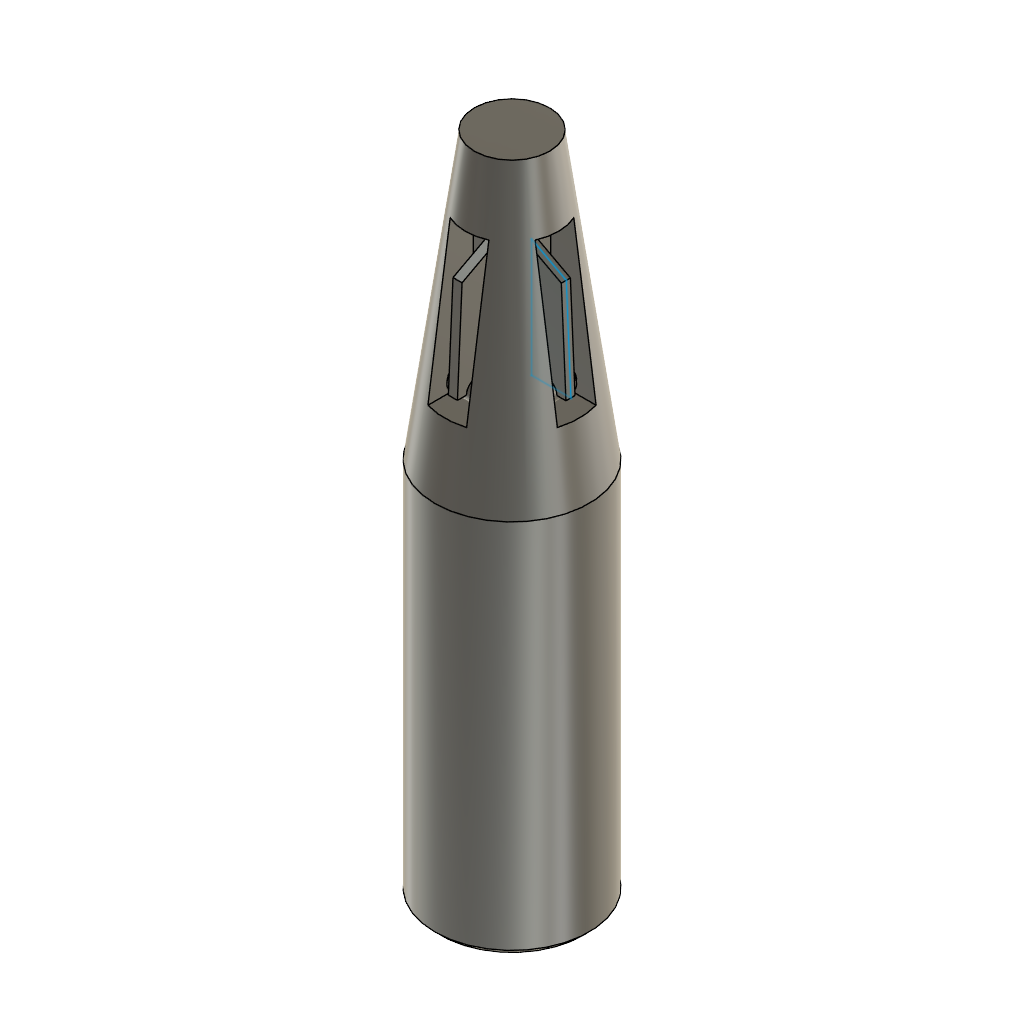
Canard Actuation Assembly (Autodesk Fusion 360 archive; units mm, degrees)
design "Canard Actuation Assembly"
part number: 2026-09-10-19-23-54-107
part number: 2026-09-14-21-49-10-628
part number: 2026-09-14-21-49-10-651
part number: 2026-09-14-21-49-10-660
part number: 2026-09-14-21-49-10-667
part number: 2026-09-14-21-49-10-675
part number: 2026-09-14-21-49-10-684
part number: 2026-09-14-21-49-10-692
part number: 2026-09-14-21-49-10-700
part number: 2026-09-14-21-49-10-708
Autodesk Fusion 360 part; units mm, degrees
note: some values were not read from the file. Chosen so that the rebuilt part matches the saved one: which bodies a step acts on.
sketch "Sketch1" plane through (0, 0, 0) normal (1, 0, 0) x (0, 1, 0)
  line L0 (0, 0) -> (0, -124.7)
  line L1 (0, -124.7) -> (25.5, -124.7)
  line L2 (25.5, -124.7) -> (25.5, 0)
  line L3 (25.5, 0) -> (12.465, 94.3539)
  line L4 (12.465, 94.3539) -> (0, 94.3539)
  line L5 (0, 94.3539) -> (0, 0)
  dimension "d5" = 124.7
  dimension "d6" = 25.5
  dimension "d7" = 124.7
  dimension "d8" = 95.25
  constraint coincident L0.start L5.end
  constraint vertical L0
  constraint perpendicular L0 L1
  constraint perpendicular L1 L2
  constraint horizontal L4
  constraint perpendicular L4 L5
  measures "d5" distance of L0.start L0.end
  measures "d6" distance of L0.end L1.end
  measures "d7" distance of L1.end L2.end
  measures "d8" distance of L2.end L3.end
revolve "Revolve1" add sketch "Sketch1" angle 360 about axis through (0, 0, 0) along (0, 0, -1) makes body 1
sketch "Sketch2" plane through (0, 0, 0) normal (0, 1, 0) x (1, 0, 0)
  line L0 (-6.3965, -72.9001) -> (5.4277, -72.9001)
  line L1 (5.4277, -72.9001) -> (5.4277, -22.9001)
  line L2 (5.4277, -22.9001) -> (-6.3965, -22.9001)
  line L3 (-6.3965, -22.9001) -> (-6.3965, -72.9001)
  dimension "d10" = 50
  constraint horizontal L0
  constraint vertical L1
  constraint horizontal L2
  constraint vertical L3
  measures "d10" distance of L0.start L2.end
extrude "Extrude1" cut sketch "Sketch2" along normal mid plane 60 bodies 1
pattern_circular "C-Pattern1" count 4 over 360 about axis through (0, 0, 0) along (0, 0, -1) of "Extrude1"
sketch "Sketch4" plane through (0, 0, 0) normal (0, 1, 0) x (1, 0, 0)
  line L0 (6.455, -27.1919) -> (6.455, -66.1919)
  line L1 (6.455, -66.1919) -> (17.9112, -60.1005)
  line L2 (17.9112, -60.1005) -> (19.4375, -27.1919)
  line L3 (19.4375, -27.1919) -> (6.455, -27.1919)
  dimension "d16" = 39
  dimension "d17" = 62
  constraint vertical L0
  constraint perpendicular L0 L3
  measures "d16" distance of L0.start L0.end
  measures "d17" angle of L0 L1
extrude "Extrude2" add sketch "Sketch4" along normal mid plane 3 separate body makes body 2
sketch "Sketch6" plane through (0, 0, 0) normal (0, 1, 0) x (1, 0, 0)
  line L0 (17.4442, -27.1976) -> (12.9542, -27.1976)
  circle A0 centre (12.9542, -27.1976) radius 3.5
  dimension "d25" = 4.49
  dimension "d26" = 7
  constraint horizontal L0
  constraint coincident L0.end A0.centre
  measures "d25" distance of L0.start L0.end
  measures "d26" diameter of A0
extrude "Extrude4" add sketch "Sketch6" along normal mid plane 10 bodies 2
chamfer "Chamfer1" distance 2 angle 45 1 faces at (-6.6456, 4.0293, -124.7) on bodies 1
sketch "Sketch9" plane through (0, -5, 0) normal (0, -1, 0) x (1, 0, 0)
  circle A0 centre (12.9542, 27.1976) radius 3.5
  circle A1 centre (12.9542, 27.1976) radius 1.5
  dimension "d44" = 3
  constraint concentric A0 A1
  measures "d44" diameter of A1
extrude "Extrude7" add sketch "Sketch9" along normal blind 4 and the other way blind 14 separate body contours A1 makes body 3
sketch "Sketch10" plane through (0, -5, 0) normal (0, -1, 0) x (1, 0, 0)
  circle A0 centre (12.9542, 27.1976) radius 3.5
  circle A1 centre (12.9542, 27.1976) radius 2
  dimension "d49" = 4
  constraint concentric A0 A1
  measures "d49" diameter of A1
pattern_circular "C-Pattern5" count 4 over 360 about axis through (0, 0, 0) along (0, 0, -1) of bodies 2 3 makes body 4 at (-1.5, -12.0128, 52.2489) makes body 5 at (-12.0128, 1.5, 52.2489) makes body 6 at (1.5, 12.0128, 52.2489) makes body 7 at (4.3333, -11.4617, 27.0482) makes body 8 at (-14.4468, -4.3333, 27.0482) makes body 9 at (0.3333, 14.4524, 27.1228)
sketch "Sketch12" plane through (-9, 0, 0) normal (-1, 0, 0) x (0, -1, 0)
  circle A0 centre (12.9542, 27.1976) radius 1.5
  circle A1 centre (12.9542, 27.1976) radius 2
  dimension "d61" = 4
  constraint concentric A0 A1
  measures "d61" diameter of A1
extrude "Extrude11" cut sketch "Sketch12" along normal blind 0 and the other way blind 24 bodies 1
pattern_circular "C-Pattern6" count 4 over 360 about axis through (0, 0, 0) along (0, 0, -1) of "Extrude11"
copy_body "Body->Comp1" bodies 1 removing the originals makes body 10 in component "Component"
copy_body "Body->Comp2" bodies 2 removing the originals makes body 11 in component "Canard_Fin1"
copy_body "Body->Comp3" bodies 4 removing the originals makes body 12 in component "Canard_Fin1 (1)"
copy_body "Body->Comp4" bodies 5 removing the originals makes body 13 in component "Canard_Fin1 (2)"
copy_body "Body->Comp5" bodies 3 removing the originals makes body 14 in component "Hinge_Pin1"
copy_body "Body->Comp6" bodies 9 removing the originals makes body 15 in component "Hinge_Pin4"
copy_body "Body->Comp7" bodies 6 removing the originals makes body 16 in component "Canard_Fin1 (3)"
copy_body "Body->Comp8" bodies 8 removing the originals makes body 17 in component "Hinge_Pin3"
copy_body "Body->Comp9" bodies 7 removing the originals makes body 18 in component "Hinge_Pin2"
component "Component" placed x (1, 0, 0) y (0, 1, 0) z (0, 0, 1) at (0, 0, 0)
component "Canard_Fin1" placed x (1, 0, 0) y (0, 1, 0) z (0, 0, 1) at (0, -0.1035, 0)
component "Canard_Fin1 (1)" placed x (1, 0, 0) y (0, 1, 0) z (0, 0, 1) at (-0.1035, 0, 0)
component "Canard_Fin1 (2)" placed x (1, 0, 0) y (0, 1, 0) z (0, 0, 1) at (0, 0.1035, 0)
component "Hinge_Pin1" placed x (1, 0, 0) y (0, 1, 0) z (0, 0, 1) at (0, 0, 0)
component "Hinge_Pin4" placed x (1, 0, 0) y (0, 1, 0) z (0, 0, 1) at (0, 0, 0)
component "Canard_Fin1 (3)" placed x (1, 0, 0) y (0, 1, 0) z (0, 0, 1) at (0.1035, 0, 0)
component "Hinge_Pin3" placed x (1, 0, 0) y (0, 1, 0) z (0, 0, 1) at (0, 0, 0)
component "Hinge_Pin2" placed x (1, 0, 0) y (0, 1, 0) z (0, 0, 1) at (0, 0, 0)
named bodies: "Canard_Fin1", "Hinge_Pin1", "Canard_Fin1 (1)", "Canard_Fin1 (2)", "Canard_Fin1 (3)", "Hinge_Pin2", "Hinge_Pin3", "Hinge_Pin4"
